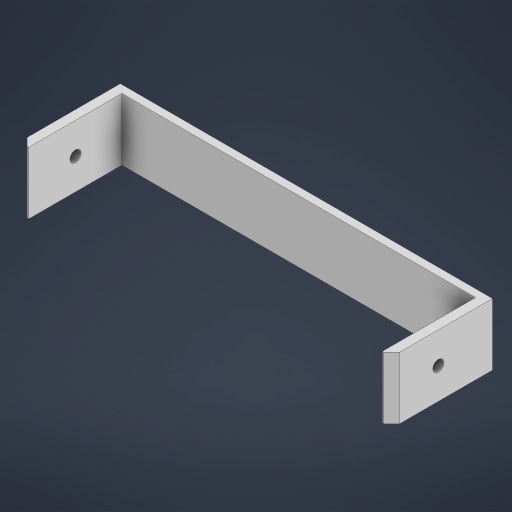
# Autodesk Inventor part: New_Arm_Brace
Saved by Autodesk Inventor 2023 (Build 270158000, 158)
## iProperties
Created: 2024-02-19
Part Number: New_Arm_Brace
Material: Generic
Document SubType Name: Modeling
Designer: kelle
Density: 1 g/cm^3
Appearance: Default
Author: kelle
Autodesk Inventor part; units mm, degrees
ref_plane "YZ Plane" through (0, 0, 0) normal (1, 0, 0) x (0, 1, 0)
ref_plane "XZ Plane" through (0, 0, 0) normal (0, 1, 0) x (-1, 0, 0)
ref_plane "XY Plane" through (0, 0, 0) normal (0, 0, 1) x (1, 0, 0)
sketch "Sketch1" plane through (0, 0, 0) normal (0, 0, 1) x (1, 0, 0)
  line L0 (76.2, -12.7) -> (-76.2, -12.7)
  line L1 (-76.2, -12.7) -> (-76.2, 12.7)
  line L2 (-76.2, 12.7) -> (76.2, 12.7)
  line L3 (76.2, 12.7) -> (76.2, -12.7)
  line L4 (76.2, -12.7) -> (-76.2, 12.7) construction
  line L5 (-76.2, -12.7) -> (76.2, 12.7) construction
  line L6 (-76.2, 12.7) -> (-72.39, 12.7)
  line L7 (-72.39, 12.7) -> (-72.39, -12.7)
  line L8 (-72.39, -12.7) -> (-76.2, -12.7)
  line L9 (-76.2, -12.7) -> (-76.2, 12.7)
  line L10 (76.2, 12.7) -> (72.39, 12.7)
  line L11 (72.39, 12.7) -> (72.39, -12.7)
  line L12 (72.39, -12.7) -> (76.2, -12.7)
  line L13 (76.2, -12.7) -> (76.2, 12.7)
  point P0 (0, 0)
  dimension "d0" = 152.4
  dimension "d1" = 25.4
  dimension "d2" = 3.81
  dimension "d3" = 3.81
  constraints: 28 end point, 6 parallel, 3 horizontal, 3 perpendicular, 2 midpoint, 2 point on line
  measures "d0" distance of L1.end L2.end
  measures "d1" distance of L0.end L1.end
  measures "d2" distance of L7.end L8.end
  measures "d3" distance of L12.end L11.end
extrude "Extrusion1" add sketch "Sketch1" along normal blind 3.175 contours L0 L7 L2 L11
extrude "Extrusion2" add sketch "Sketch1" along normal blind 41.275 contours L0 L11 L2 L3 | L0 L1 L2 L7
chamfer "Chamfer1" distance 3.175 angle 45 2 edges at (-76.2, 0, 41.275) (76.2, 0, 41.275)
sketch "Sketch2" plane through (76.2, -12.7, 0) normal (1, 0, 0) x (0, 0, -1)
  line L0 (-3.175, 25.4) -> (-41.275, 25.4) construction
  line L1 (-22.225, 25.4) -> (-22.225, 0) construction
  line L2 (0, 0) -> (-38.1, 0) construction
  line L3 (-41.275, 0) -> (-41.275, 25.4) construction
  line L4 (-41.275, 12.7) -> (0, 12.7) construction
  circle A0 centre (-22.225, 12.7) radius 2.25
  line L5 (-3.175, 0) -> (-3.175, 25.4) projected
  dimension "d11" = 4.5
  dimension "d14" = 19.05
  constraints: 4 end point, 3 midpoint, 2 point on line, 1 centre point, 1 horizontal, 1 vertical
  measures "d11" diameter of A0
  measures "d14" distance from line of L5 A0.centre
extrude "Extrusion3" cut sketch "Sketch2" against normal through all
body "Solid1"
